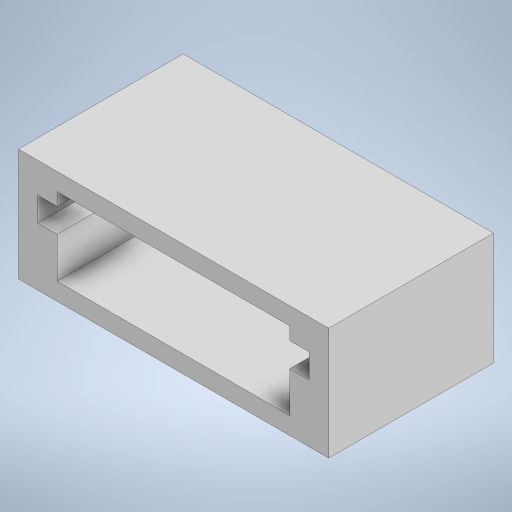
# Autodesk Inventor part: jst - 1 mm 6 pin female
Saved by Autodesk Inventor 2024 (Build 280153000, 153)
## iProperties
Created: 2023-10-20
Part Number: jst - 1 mm 6 pin female
Material: Všeobecné
Document SubType Name: Modeling
Designer: jaryj
Density: 1 g/cm^3
Appearance: Výchozí
Author: jaryj
Autodesk Inventor part; units mm, degrees
ref_plane "YZ Plane" through (0, 0, 0) normal (1, 0, 0) x (0, 1, 0)
ref_plane "XZ Plane" through (0, 0, 0) normal (0, 1, 0) x (-1, 0, 0)
ref_plane "XY Plane" through (0, 0, 0) normal (0, 0, 1) x (1, 0, 0)
sketch "Náčrt1" plane through (0, 0, 0) normal (0, 0, 1) x (1, 0, 0)
  line L0 (-4, 1.45) -> (4, 1.45)
  line L1 (4, 1.45) -> (4, -1.45)
  line L2 (4, -1.45) -> (-4, -1.45)
  line L3 (-4, -1.45) -> (-4, 1.45)
  line L4 (-4, 1.45) -> (4, -1.45) construction
  line L5 (4, 1.45) -> (-4, -1.45) construction
  line L6 (-3, 1) -> (3, 1)
  line L7 (3, 1) -> (3, -1)
  line L8 (3, -1) -> (-3, -1)
  line L9 (-3, -1) -> (-3, 1)
  line L10 (-3, 1) -> (3, -1) construction
  line L11 (3, 1) -> (-3, -1) construction
  line L12 (-3, 0.67) -> (-3.5, 0.67)
  line L13 (-3.5, 0.67) -> (-3.5, 0.05)
  line L14 (-3.5, 0.05) -> (-3, 0.05)
  line L15 (3, 0.67) -> (3.5, 0.67)
  line L16 (3.5, 0.67) -> (3.5, 0.05)
  line L17 (3.5, 0.05) -> (3, 0.05)
  point P0 (0, 0)
  dimension "d0" = 8
  dimension "d1" = 2.9
  dimension "d2" = 2
  dimension "d3" = 6
  dimension "d4" = 7
  dimension "d5" = 0.62
  dimension "d6" = 1.5
  constraints: 36 end point, 8 perpendicular, 4 midpoint, 4 parallel, 4 point on line, 2 equal length, 2 horizontal, 1 horizontal alignment
  measures "d0" distance of L0.start L0.end
  measures "d1" distance of L0.end L1.end
  measures "d2" distance between parallel lines of L6 L8
  measures "d3" distance of L6.start L6.end
  measures "d4" distance between parallel lines of L16 L13
  measures "d5" distance between parallel lines of L14 L12
  measures "d6" distance between parallel lines of L2 L17
extrude "Vysunutí1" add sketch "Náčrt1" along normal blind 4.25
extrude "Vysunutí2" add sketch "Náčrt1" along normal blind 1.25 contours L6 L7 L8 L9 | L9 L14 L13 L12 | L15 L16 L17 L7
sketch "Náčrt2" plane through (0, 0, 1.25) normal (0, 0, 1) x (1, 0, 0)
  line L0 (-2.65, 0.67) -> (-2.35, 0.67)
  line L1 (-2.35, 0.67) -> (-2.35, 0.37)
  line L2 (-2.35, 0.37) -> (-2.65, 0.37)
  line L3 (-2.65, 0.37) -> (-2.65, 0.67)
  line L4 (-2.65, 0.67) -> (-2.35, 0.37) construction
  line L5 (-2.35, 0.67) -> (-2.65, 0.37) construction
  line L6 (-1.65, 0.67) -> (-1.35, 0.67)
  line L7 (-1.35, 0.67) -> (-1.35, 0.37)
  line L8 (-1.35, 0.37) -> (-1.65, 0.37)
  line L9 (-1.65, 0.37) -> (-1.65, 0.67)
  line L10 (-1.65, 0.67) -> (-1.35, 0.37) construction
  line L11 (-1.35, 0.67) -> (-1.65, 0.37) construction
  line L12 (-0.65, 0.67) -> (-0.35, 0.67)
  line L13 (-0.35, 0.67) -> (-0.35, 0.37)
  line L14 (-0.35, 0.37) -> (-0.65, 0.37)
  line L15 (-0.65, 0.37) -> (-0.65, 0.67)
  line L16 (-0.65, 0.67) -> (-0.35, 0.37) construction
  line L17 (-0.35, 0.67) -> (-0.65, 0.37) construction
  line L18 (0.35, 0.67) -> (0.65, 0.67)
  line L19 (0.65, 0.67) -> (0.65, 0.37)
  line L20 (0.65, 0.37) -> (0.35, 0.37)
  line L21 (0.35, 0.37) -> (0.35, 0.67)
  line L22 (0.35, 0.67) -> (0.65, 0.37) construction
  line L23 (0.65, 0.67) -> (0.35, 0.37) construction
  line L24 (1.35, 0.67) -> (1.65, 0.67)
  line L25 (1.65, 0.67) -> (1.65, 0.37)
  line L26 (1.65, 0.37) -> (1.35, 0.37)
  line L27 (1.35, 0.37) -> (1.35, 0.67)
  line L28 (1.35, 0.67) -> (1.65, 0.37) construction
  line L29 (1.65, 0.67) -> (1.35, 0.37) construction
  line L30 (2.35, 0.67) -> (2.65, 0.67)
  line L31 (2.65, 0.67) -> (2.65, 0.37)
  line L32 (2.65, 0.37) -> (2.35, 0.37)
  line L33 (2.35, 0.37) -> (2.35, 0.67)
  line L34 (2.35, 0.67) -> (2.65, 0.37) construction
  line L35 (2.65, 0.67) -> (2.35, 0.37) construction
  line L36 (-3, -1) -> (-3, 0.05) projected
  line L37 (-3, 0.37) -> (-2.65, 0.37) construction
  line L38 (2.65, 0.37) -> (3, 0.37) construction
  line L39 (3, 0.05) -> (3, -1) construction
  point P0 (0, 0)
  point P1 (-2.5, 0.52)
  point P2 (-1.5, 0.52)
  point P3 (-0.5, 0.52)
  point P4 (0.5, 0.52)
  point P5 (1.5, 0.52)
  point P6 (2.5, 0.52)
  point P7 (-3, 0.67)
  dimension "d13" = 1
  dimension "d19" = 0.3
  dimension "d20" = 0.3
  constraints: 76 end point, 3 point on line, 2 collinear, 2 horizontal, 2 midpoint, 2 parallel, 2 perpendicular, 1 coincident, 1 horizontal alignment, 54 other
  measures "d13" distance of L0.start L6.start
  measures "d19" distance of L1.end L2.end
  measures "d20" distance of L0.end L1.end
extrude "Vysunutí3" add sketch "Náčrt2" along normal blind 2
